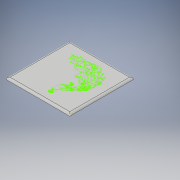
# Autodesk Inventor part: Card_1
Saved by Autodesk Inventor 2019.4 (Build 234330000, 330)
## iProperties
Created: 2020-03-24
Part Number: Card_1
Material: Generic
Document SubType Name: Modeling
Designer: Jorian Brusind
Density: 1 g/cm^3
Appearance: Default
Author: Jorian Brusind
Autodesk Inventor part; units mm, degrees
(part 1 of 2)
ref_plane "YZ Plane" through (0, 0, 0) normal (1, 0, 0) x (0, 1, 0)
ref_plane "XZ Plane" through (0, 0, 0) normal (0, 1, 0) x (-1, 0, 0)
ref_plane "XY Plane" through (0, 0, 0) normal (0, 0, 1) x (1, 0, 0)
sketch "Sketch1" plane through (0, 0, 0) normal (0, 1, 0) x (-1, 0, 0)
  line L0 (0, 0) -> (80, 0)
  line L1 (80, 0) -> (80, -80)
  line L2 (80, -80) -> (0, -80)
  line L3 (0, -80) -> (0, 0)
  line L4 (70, -70) -> (70, -10)
  line L5 (70, -10) -> (10, -10)
  line L6 (10, -10) -> (10, -70)
  line L7 (10, -70) -> (70, -70)
  dimension "d0" = 80
  dimension "d1" = 80
  dimension "d2" = 10
  constraints: 16 end point, 4 parallel, 2 perpendicular, 1 horizontal, 3 other
  measures "d0" distance of L1.end L2.end
  measures "d1" distance of L0.end L1.end
  measures "d2" distance between parallel lines of L1 L4
extrude "Extrusion1" add sketch "Sketch1" along normal blind 2.5
fillet "Fillet1" radius 2.5 4 edges at (-40, 2.5, 0) (0, 2.5, -40) (-40, 2.5, -80) (-80, 2.5, -40)
sketch "Sketch2" plane through (0, 2.5, 0) normal (0, 1, 0) x (1, 0, 0)
  line L0 (-70, 70) -> (-70, 10) projected
  line L1 (-70, 10) -> (-10, 10) projected
  line L2 (-70, 70) -> (-10, 70)
  line L3 (-10, 70) -> (-10, 10)
  line L4 (-10, 10) -> (-70, 10)
  line L5 (-70, 10) -> (-70, 70)
  point P0 (0, 0)
  constraints: 8 end point, 2 parallel, 1 horizontal, 1 perpendicular
extrude "Extrusion2" add sketch "Sketch2" against normal blind 1
sketch "Sketch3" plane through (0, 1.5, 0) normal (0, -1, 0) x (1, 0, 0)
  line L0 (-63.3517, -10.3054) -> (-12.5932, -10.3054) construction
  line L1 (-12.5932, -10.3054) -> (-12.5932, -69.5003) construction
  line L2 (-12.5932, -69.5003) -> (-63.3517, -69.5003) construction
  line L3 (-63.3517, -69.5003) -> (-63.3517, -10.3054) construction
  circle A0 centre (-36.5711, -14.8755) radius 0.2923
  spline S0 degree 4 poles (-35.324, -13.1457) (-35.5446, -13.3836) (-34.7422, -13.6925) (-35.8936, -14.24) (-35.5511, -14.8191) (-35.9597, -15.77) (-36.825, -15.6199) (-37.3254, -15.6398) knots 0 0 0 0 0 0.31317 0.445072 0.586813 1 1 1 1 1
  spline S1 degree 4 poles (-37.3254, -15.6398) (-37.2583, -15.4035) (-36.9842, -15.1648) (-37.3716, -13.9172) (-35.5713, -13.5514) (-35.7305, -13.4977) (-36.1286, -13.2161) knots 0 0 0 0 0 0.420009 0.598576 1 1 1 1 1
  spline S2 degree 4 poles (-36.1286, -13.2161) (-36.1977, -13.1672) (-36.3236, -13.3314) (-37.1252, -12.6262) (-37.6158, -14.3916) (-38.3336, -14.3814) (-38.1098, -15.4286) knots 0 0 0 0 0 0.20425 0.384643 1 1 1 1 1
  spline S3 degree 3 poles (-38.9144, -17.1685) (-39.2781, -16.9978) (-37.8451, -15.6043) (-38.1098, -15.4286) knots 0 0 0 0 1 1 1 1
  spline S4 degree 4 poles (-38.9144, -17.1685) (-38.8152, -17.5134) (-37.7404, -15.2772) (-37.1183, -18.5822) (-34.1569, -13.527) (-35.4039, -17.8434) (-35.7063, -17.3998) knots 0 0 0 0 0 0.380958 0.551634 1 1 1 1 1
  spline S5 degree 4 poles (-35.324, -13.1457) (-35.5269, -12.7152) (-30.8309, -14.436) (-33.9129, -18.4293) (-33.8615, -18.3326) knots 0 0 0 0 0 1 1 1 1 1
  spline S6 degree 4 poles (-33.8615, -18.3326) (-35.1288, -18.3656) (-31.8331, -20.408) (-33.8396, -20.6327) (-27.0068, -23.04) (-26.7008, -23.4984) (-25.4635, -25.0323) (-25.2341, -25.4897) knots 0 0 0 0 0 0.314732 0.481412 0.642299 1 1 1 1 1
  spline S7 degree 4 poles (-25.2341, -25.4897) (-25.4023, -25.6156) (-25.7938, -24.9389) (-27.0573, -23.6199) (-30.4827, -22.3618) (-31.9985, -23.0805) (-32.4743, -21.943) (-37.6197, -21.044) (-37.7605, -24.854) (-36.5634, -26.7006) (-35.7063, -26.8823) knots 0 0 0 0 0 0.17093 0.27416 0.381186 0.49379 0.600301 0.71651 1 1 1 1 1
  spline S8 degree 4 poles (-35.7063, -26.8823) (-35.4306, -26.8662) (-35.7103, -27.6356) (-37.8889, -26.2872) (-36.9937, -25.7229) (-38.9297, -25.107) (-37.7887, -22.8322) (-39.896, -21.88) (-38.051, -17.7127) (-36.0866, -18.5751) (-35.7063, -17.3998) knots 0 0 0 0 0 0.15712 0.241782 0.341646 0.440215 0.558312 0.68699 1 1 1 1 1
  spline S9 degree 5 poles (-33.3611, -22.4991) (-33.2761, -22.525) (-33.1323, -22.7463) (-33.0805, -23.4713) (-31.2722, -23.0711) (-30.0002, -22.6532) (-27.8482, -26.1645) (-29.0106, -24.5854) (-29.6261, -24.0335) (-30.7533, -23.6216) (-31.6668, -24.1266) (-33.7566, -23.2068) (-33.5906, -22.5757) (-33.4394, -22.4753) (-33.3611, -22.4991) knots 0 0 0 0 0 0 0.106127 0.195486 0.298213 0.408816 0.518685 0.625012 0.727572 0.824846 0.902338 1 1 1 1 1 1
  spline S10 degree 4 poles (-34.5544, -27.0158) (-34.756, -26.8509) (-32.4655, -27.7887) (-33.815, -25.1287) (-31.1635, -27.2727) (-31.4203, -24.5805) (-29.3028, -26.5518) (-30.6351, -24.5794) (-28.6311, -25.5338) knots 0 0 0 0 0 0.293192 0.431361 0.562283 0.684411 1 1 1 1 1
  spline S11 degree 4 poles (-28.6311, -25.5338) (-28.4787, -25.3926) (-28.0839, -26.0174) (-29.7828, -25.7606) (-29.7026, -26.1515) (-30.1461, -26.5172) (-30.7038, -26.0429) (-30.8578, -26.9801) (-31.5435, -26.9955) (-31.992, -27.4243) (-32.6157, -26.6422) (-32.7974, -28.0141) (-33.9737, -27.5055) (-34.4403, -27.4572) (-34.5544, -27.0158) knots 0 0 0 0 0 0.143761 0.210775 0.282047 0.347044 0.419443 0.494672 0.570855 0.64562 0.720443 0.799389 1 1 1 1 1
  spline S12 degree 3 poles (-32.3859, -20.0818) (-31.8556, -19.6395) (-27.7329, -20.2333) (-26.6799, -22.7987) knots 0 0 0 0 1 1 1 1
  spline S13 degree 4 poles (-32.3859, -20.0818) (-32.544, -20.1533) (-29.582, -22.2131) (-29.798, -20.0561) (-26.6184, -23.2562) (-26.6799, -22.7987) knots 0 0 0 0 0 0.510331 1 1 1 1 1
  spline S14 degree 4 poles (-35.9258, -27.4345) (-35.5506, -27.1339) (-35.543, -28.1757) (-33.3169, -27.6119) (-32.9054, -28.5495) (-32.099, -29.7207) (-30.6072, -30.9729) (-29.9615, -30.1066) (-29.5156, -30.5716) knots 0 0 0 0 0 0.273602 0.406043 0.548907 0.683354 1 1 1 1 1
  spline S15 degree 4 poles (-29.5156, -30.5716) (-29.2202, -30.6478) (-30.1433, -31.6427) (-30.3254, -30.3824) (-31.1214, -31.3006) (-30.8679, -31.6024) (-30.842, -32.4055) (-30.1008, -32.916) (-30.8967, -33.4395) (-30.1082, -33.9699) (-29.7346, -34.3371) knots 0 0 0 0 0 0.231424 0.328427 0.428678 0.530661 0.628034 0.725923 1 1 1 1 1
  spline S16 degree 4 poles (-29.7346, -34.3371) (-29.3878, -34.6781) (-30.3659, -34.1189) (-30.4227, -34.2157) (-31.503, -34.2428) (-31.5893, -34.4521) (-33.027, -35.5237) (-32.9708, -34.6703) (-31.8667, -34.1719) (-32.5619, -34.097) (-32.7749, -34.3573) (-33.9131, -34.6609) (-33.5335, -33.9376) (-33.0108, -34.1956) (-32.4249, -33.8451) (-32.9337, -33.674) (-33.706, -33.5322) (-32.7473, -33.2202) (-32.3814, -33.4344) (-31.5548, -33.5668) (-31.3728, -33.9075) (-31.1352, -33.3806) knots 0 0 0 0 0 0.102598 0.152726 0.207977 0.263777 0.320477 0.373024 0.41872 0.467777 0.51215 0.561575 0.609015 0.651576 0.696303 0.740357 0.785856 0.834092 0.882144 1 1 1 1 1
  spline S17 degree 4 poles (-31.1352, -33.3806) (-31.1314, -33.1006) (-31.0926, -32.3796) (-31.5407, -32.0448) (-31.6958, -30.9795) knots 0 0 0 0 0 1 1 1 1 1
  spline S18 degree 4 poles (-31.6958, -30.9795) (-31.666, -30.9185) (-32.9258, -29.9607) (-33.0237, -28.6807) (-34.4784, -28.818) (-36.393, -27.4471) (-35.9258, -27.4345) knots 0 0 0 0 0 0.400646 0.601925 1 1 1 1 1
  spline S19 degree 4 poles (-32.5781, -28.1533) (-32.0733, -28.1334) (-32.5286, -29.7003) (-28.3942, -29.6937) (-27.0116, -29.0351) (-27.4794, -30.2319) knots 0 0 0 0 0 0.455262 1 1 1 1 1
  spline S20 degree 4 poles (-32.5781, -28.1533) (-32.752, -28.8754) (-30.7966, -29.9892) (-29.2732, -30.7108) (-27.4794, -30.2319) knots 0 0 0 0 0 1 1 1 1 1
  spline S21 degree 3 poles (-31.9981, -27.8266) (-31.3048, -28.2374) (-30.1278, -28.9395) (-28.02, -28.4008) knots 0 0 0 0 1 1 1 1
  spline S22 degree 3 poles (-31.9981, -27.8266) (-32.159, -28.3516) (-29.309, -29.8112) (-26.2551, -28.9797) knots 0 0 0 0 1 1 1 1
  spline S23 degree 3 poles (-28.02, -28.4008) (-27.4223, -28.5754) (-26.0857, -27.8191) (-26.2551, -28.9797) knots 0 0 0 0 1 1 1 1
  spline S24 degree 5 poles (-30.8304, -27.4166) (-30.8198, -27.3784) (-30.735, -27.3314) (-30.4283, -27.377) (-30.3728, -27.806) (-29.4819, -27.5359) (-28.6522, -28.0829) (-26.9449, -27.1371) (-26.9592, -28.3103) (-27.5005, -27.9622) (-28.3391, -28.2269) (-29.6001, -27.9856) (-29.9402, -28.0264) (-30.7153, -27.6691) (-30.8488, -27.4824) (-30.8304, -27.4166) knots 0 0 0 0 0 0 0.06847 0.134935 0.226492 0.320983 0.41447 0.511985 0.607211 0.700225 0.797172 0.882041 1 1 1 1 1 1
  spline S25 degree 5 poles (-29.6277, -27.2599) (-29.6131, -27.1962) (-29.3962, -27.1169) (-28.6593, -27.1471) (-28.6951, -27.3926) (-26.953, -26.1162) (-27.3022, -26.7784) (-25.8648, -27.2556) (-26.7786, -27.9342) (-26.8765, -27.0905) (-27.6032, -27.0829) (-28.3562, -27.7093) (-29.4112, -27.4986) (-29.6452, -27.3368) (-29.6277, -27.2599) knots 0 0 0 0 0 0 0.117746 0.200054 0.303318 0.403009 0.497632 0.581512 0.677264 0.774 0.857863 1 1 1 1 1 1
  spline S26 degree 5 poles (-28.9567, -26.8367) (-28.8039, -26.8311) (-28.3186, -26.542) (-27.1771, -25.5262) (-25.4527, -27.3948) (-24.9989, -26.5696) (-26.8849, -25.2773) (-28.7538, -25.9258) (-29.1284, -26.6777) (-29.0748, -26.841) (-28.9567, -26.8367) knots 0 0 0 0 0 0 0.223292 0.365456 0.553127 0.712011 0.827339 1 1 1 1 1 1
  spline S27 degree 5 poles (-25.2341, -24.8772) (-25.2139, -24.9767) (-25.0028, -25.1808) (-24.3449, -25.5142) (-25.0904, -26.3444) (-23.5868, -25.9629) (-22.7451, -26.6919) (-21.7421, -27.7341) (-22.2449, -26.4551) (-23.5022, -25.9794) (-23.9866, -24.5416) (-25.0568, -24.5977) (-25.2586, -24.7561) (-25.2341, -24.8772) knots 0 0 0 0 0 0 0.119065 0.209319 0.316618 0.415827 0.527874 0.652848 0.762595 0.855295 1 1 1 1 1 1
  spline S28 degree 3 poles (-23.9961, -26.7161) (-22.4627, -27.8802) (-20.8684, -31.6059) (-18.6876, -30.7743) knots 0 0 0 0 1 1 1 1
  spline S29 degree 4 poles (-23.9961, -26.7161) (-23.918, -26.6354) (-22.7506, -26.261) (-21.1004, -29.3277) (-20.4862, -29.8276) (-19.4071, -30.9349) (-18.4206, -30.3496) (-18.6876, -30.7743) knots 0 0 0 0 0 0.362224 0.54379 0.715209 1 1 1 1 1
  spline S30 degree 5 poles (-23.9961, -27.4166) (-24.0084, -27.3157) (-23.7565, -27.4117) (-22.6333, -28.3225) (-21.0445, -30.8303) (-20.9846, -30.4847) (-22.2092, -31.6756) (-21.8204, -30.0675) (-22.8853, -29.6975) (-22.7683, -28.9575) (-23.686, -27.943) (-23.9837, -27.5186) (-23.9961, -27.4166) knots 0 0 0 0 0 0 0.168899 0.268082 0.386273 0.508516 0.61038 0.728446 0.829264 1 1 1 1 1 1
  spline S31 degree 3 poles (-24.0993, -28.03) (-23.4446, -28.7383) (-20.4539, -32.1956) (-23.4494, -35.6288) knots 0 0 0 0 1 1 1 1
  spline S32 degree 4 poles (-23.4494, -35.6288) (-24.264, -35.9348) (-24.9335, -34.8994) (-23.1097, -35.9947) (-21.6779, -30.0877) (-24.1929, -28.6957) (-24.0993, -28.03) knots 0 0 0 0 0 0.300614 0.469562 1 1 1 1 1
  spline S33 degree 4 poles (-25.0725, -27.5346) (-24.8746, -27.2275) (-22.7058, -29.9805) (-23.1973, -34.4136) (-26.2584, -32.3924) (-25.4951, -32.4837) (-23.7291, -31.7895) (-24.1652, -30.0658) (-23.9832, -28.6385) (-25.4514, -27.5272) (-25.0725, -27.5346) knots 0 0 0 0 0 0.306197 0.41617 0.507229 0.595458 0.6902 0.801188 1 1 1 1 1
  spline S34 degree 5 poles (-25.9194, -27.3048) (-25.9589, -27.3397) (-25.8277, -27.6124) (-25.1566, -28.4149) (-25.287, -28.3236) (-24.9688, -32.2896) (-27.6153, -30.4366) (-26.2254, -32.3751) (-25.0718, -30.9028) (-24.5869, -30.5734) (-24.0451, -29.0091) (-25.4585, -27.5295) (-25.8674, -27.2588) (-25.9194, -27.3048) knots 0 0 0 0 0 0 0.120573 0.208552 0.309906 0.418809 0.526835 0.630512 0.742533 0.841179 1 1 1 1 1 1
  ellipse E0 centre (-21.017, -31.7834) end of major axis (-21.2816, -31.2172) minor radius 0.4541
  ellipse E1 centre (-18.4895, -33.3373) end of major axis (-18.8637, -32.8075) minor radius 0.4897
  ellipse E2 centre (-21.6934, -42.4408) end of major axis (-21.1885, -41.4828) minor radius 0.8739
  ellipse E3 centre (-15.5478, -42.5952) end of major axis (-15.5478, -41.4335) minor radius 0.8581
  ellipse E4 centre (-19.3699, -49.1886) end of major axis (-18.9081, -47.7943) minor radius 1.306
  ellipse E5 centre (-27.7073, -52.7002) end of major axis (-26.5866, -51.7716) minor radius 1.2181
  ellipse E6 centre (-17.1812, -55.9206) end of major axis (-16.5391, -54.5789) minor radius 0.9936
  ellipse E7 centre (-28.8439, -61.7728) end of major axis (-27.7073, -61.3217) minor radius 0.7832
  ellipse E8 centre (-44.2997, -60.5199) end of major axis (-42.6078, -60.5199) minor radius 1.1489
  spline S35 degree 3 poles (-19.5271, -31.3956) (-19.0196, -31.8926) (-17.7371, -31.8552) (-17.9516, -31.0393) knots 0 0 0 0 1 1 1 1
  spline S36 degree 4 poles (-17.9516, -31.0393) (-17.8718, -30.4122) (-15.8826, -33.3458) (-19.1868, -32.8117) (-19.5271, -31.3956) knots 0 0 0 0 0 1 1 1 1 1
  spline S37 degree 4 poles (-20.8379, -34.6217) (-19.4947, -34.9164) (-21.2318, -32.5629) (-17.6677, -33.2688) (-20.3107, -30.9795) knots 0 0 0 0 0 1 1 1 1 1
  spline S38 degree 4 poles (-20.3107, -30.9795) (-20.6685, -30.6769) (-20.6934, -31.3689) (-19.9364, -31.3263) (-20.195, -32.8112) (-20.9449, -32.9065) (-21.6592, -32.7466) (-21.7848, -31.827) (-21.907, -31.6466) knots 0 0 0 0 0 0.267734 0.396357 0.532031 0.670594 1 1 1 1 1
  spline S39 degree 4 poles (-21.907, -31.6466) (-22.3419, -31.4487) (-20.8709, -33.7898) (-21.5359, -33.7291) (-21.2111, -34.7898) (-20.8379, -34.6217) knots 0 0 0 0 0 0.51757 1 1 1 1 1
  spline S40 degree 4 poles (-20.766, -35.1172) (-19.8876, -34.9373) (-20.1572, -33.9627) (-19.4524, -34.5635) (-19.7247, -36.2501) (-20.5302, -36.787) (-21.0324, -36.7624) (-21.7811, -36.3233) (-21.8838, -35.5783) (-22.1093, -35.1229) (-21.5483, -33.5183) (-21.5122, -35.2087) (-21.2854, -35.0098) (-20.766, -35.1172) knots 0 0 0 0 0 0.182152 0.257602 0.342773 0.433832 0.515997 0.595919 0.678531 0.753704 0.825493 1 1 1 1 1
  spline S41 degree 4 poles (-19.0268, -34.0685) (-18.7409, -34.1417) (-17.1836, -35.7942) (-17.1543, -32.9167) (-17.764, -32.9276) knots 0 0 0 0 0 1 1 1 1 1
  spline S42 degree 4 poles (-17.764, -32.9276) (-17.8387, -32.6933) (-17.3458, -32.89) (-16.8285, -33.1066) (-16.4625, -33.8615) (-16.5379, -34.5141) (-16.7185, -35.0701) (-17.2038, -35.2058) (-17.6314, -35.4748) (-18.4579, -35.193) (-18.9875, -34.8196) (-19.2024, -34.218) (-19.0268, -34.0685) knots 0 0 0 0 0 0.171381 0.262578 0.355555 0.445026 0.530668 0.614709 0.701973 0.792644 1 1 1 1 1
  spline S43 degree 5 poles (-19.4194, -35.9625) (-19.295, -36.0313) (-18.9705, -36.0406) (-18.3013, -35.7473) (-19.0957, -35.6603) (-18.9284, -34.9173) (-19.3485, -34.7866) (-19.4737, -33.2171) (-19.6394, -35.2858) (-19.2948, -35.023) (-19.6406, -35.6443) (-19.5523, -35.8889) (-19.4194, -35.9625) knots 0 0 0 0 0 0 0.143801 0.239764 0.360191 0.482966 0.611681 0.742234 0.846271 1 1 1 1 1 1
  spline S44 degree 5 poles (-14.3221, -37.2251) (-14.273, -37.225) (-14.2224, -37.0537) (-14.2438, -36.3783) (-14.2395, -36.1076) (-14.5116, -35.2835) (-14.6889, -34.9296) (-15.1743, -34.5084) (-15.5757, -34.3933) (-16.2251, -34.3778) (-16.6103, -34.6493) (-15.7195, -35.1067) (-15.4355, -35.1895) (-14.7936, -36.0142) (-14.7853, -36.1341) (-14.5112, -37.0079) (-14.3779, -37.2252) (-14.3221, -37.2251) knots 0 0 0 0 0 0 0.092663 0.155941 0.233987 0.313281 0.389538 0.457583 0.525214 0.594431 0.66685 0.742099 0.825589 0.894681 1 1 1 1 1 1
  spline S45 degree 5 poles (-16.4214, -35.3061) (-16.4018, -35.2543) (-16.2185, -35.2898) (-15.5483, -35.7263) (-15.4414, -36.4002) (-14.5668, -37.0976) (-13.8258, -38.4064) (-14.0517, -39.8851) (-13.261, -40.9923) (-14.3695, -42.258) (-12.1945, -43.4637) (-13.432, -43.6748) (-13.7621, -42.6858) (-14.2319, -42.0616) (-14.6289, -41.0906) (-15.0867, -39.8382) (-14.7116, -38.763) (-15.4988, -37.4661) (-15.0187, -36.9438) (-16.2114, -35.7589) (-16.45, -35.3819) (-16.4214, -35.3061) knots 0 0 0 0 0 0 0.053732 0.097834 0.156445 0.222119 0.289791 0.356859 0.415576 0.469792 0.521624 0.571562 0.623429 0.682083 0.742885 0.805694 0.870231 0.921522 1 1 1 1 1 1
  spline S46 degree 5 poles (-15.9677, -40.9926) (-15.8484, -41.0734) (-15.4979, -41.1314) (-14.658, -40.9692) (-15.504, -40.7181) (-15.1203, -39.5113) (-15.3578, -39.0368) (-15.735, -37.7705) (-15.5769, -38.0538) (-16.6952, -35.2921) (-16.4608, -36.6677) (-16.3319, -36.6643) (-16.0555, -37.7254) (-16.253, -38.0379) (-15.8485, -38.8772) (-16.2821, -39.9553) (-15.7901, -40.2184) (-16.1432, -40.7024) (-16.0829, -40.9145) (-15.9677, -40.9926) knots 0 0 0 0 0 0 0.07587 0.12937 0.197561 0.265254 0.343498 0.415321 0.482169 0.547672 0.611 0.670605 0.737417 0.806106 0.872412 0.926727 1 1 1 1 1 1
  spline S47 degree 5 poles (-17.6207, -41.3723) (-17.526, -41.4325) (-17.2108, -41.1854) (-16.3758, -39.8158) (-16.2257, -40.0312) (-16.9062, -34.882) (-17.3821, -36.4562) (-16.7825, -37.4206) (-17.3208, -38.3171) (-17.1453, -39.4507) (-17.3233, -39.9427) (-17.5615, -40.3444) (-17.719, -41.0919) (-17.6859, -41.3309) (-17.6207, -41.3723) knots 0 0 0 0 0 0 0.141772 0.233793 0.345818 0.460441 0.567888 0.654576 0.746613 0.834588 0.902411 1 1 1 1 1 1
  spline S48 degree 5 poles (-18.9081, -36.4109) (-18.8365, -36.4058) (-18.7132, -36.2971) (-18.505, -35.8809) (-18.0681, -37.0072) (-18.3049, -37.1322) (-18.62, -37.8454) (-19.0368, -37.7127) (-19.4634, -37.4155) (-19.5131, -36.9259) (-19.5161, -36.4286) (-19.2378, -36.0701) (-19.069, -36.3536) (-18.9668, -36.4151) (-18.9081, -36.4109) knots 0 0 0 0 0 0 0.122221 0.208647 0.312805 0.419979 0.526064 0.631352 0.728714 0.824557 0.89992 1 1 1 1 1 1
  spline S49 degree 5 poles (-19.868, -37.2702) (-19.7939, -37.2817) (-19.7018, -37.5036) (-19.6382, -38.2929) (-18.9612, -38.4002) (-18.6891, -38.4019) (-17.5038, -37.8134) (-18.2743, -37.0477) (-17.5089, -36.693) (-17.6449, -37.7812) (-17.2851, -37.9782) (-17.5203, -39.0215) (-18.0572, -39.4942) (-18.7508, -39.8247) (-19.5524, -39.6958) (-20.0798, -38.9816) (-20.5418, -38.6362) (-20.1437, -37.5098) (-19.9557, -37.2566) (-19.868, -37.2702) knots 0 0 0 0 0 0 0.079097 0.133351 0.199973 0.259999 0.31817 0.376815 0.434654 0.494724 0.561731 0.630756 0.701479 0.773466 0.846774 0.906384 1 1 1 1 1 1
  spline S50 degree 5 poles (-20.6923, -37.0413) (-20.7937, -37.0047) (-21.0413, -36.9685) (-21.5325, -37.0126) (-20.8933, -38.8414) (-21.5679, -38.581) (-23.2741, -41.9479) (-21.3958, -39.6024) (-21.2051, -41.2401) (-19.7575, -40.5302) (-20.431, -38.9723) (-20.3653, -38.4828) (-20.4975, -37.3272) (-20.4955, -37.1504) (-20.6075, -37.0719) (-20.6923, -37.0413) knots 0 0 0 0 0 0 0.097411 0.176594 0.273172 0.374402 0.47305 0.572074 0.667248 0.76187 0.848421 0.918566 1 1 1 1 1 1
  spline S51 degree 5 poles (-22.7021, -36.6766) (-22.6255, -36.6777) (-22.6974, -37.1269) (-23.3882, -38.9246) (-23.5146, -38.9014) (-25.1864, -40.3908) (-26.3321, -39.047) (-25.6333, -37.8786) (-25.2484, -39.3618) (-23.512, -38.3052) (-23.7144, -38.3107) (-23.0402, -37.0298) (-22.771, -36.6757) (-22.7021, -36.6766) knots 0 0 0 0 0 0 0.15502 0.255703 0.369442 0.475363 0.577682 0.674868 0.774185 0.860446 1 1 1 1 1 1
  spline S52 degree 5 poles (-25.9194, -39.9564) (-25.8568, -39.8675) (-25.6947, -39.7741) (-25.3735, -39.8915) (-25.178, -40.5024) (-24.1491, -40.6864) (-23.3894, -38.3827) (-23.1178, -39.7388) (-23.788, -40.0679) (-24.3296, -41.0394) (-25.1127, -41.0528) (-25.8923, -40.9387) (-26.0618, -40.3521) (-25.9966, -40.0659) (-25.9194, -39.9564) knots 0 0 0 0 0 0 0.097167 0.178472 0.272394 0.374095 0.481458 0.588908 0.688995 0.795073 0.880225 1 1 1 1 1 1
  spline S53 degree 5 poles (-23.6773, -40.4903) (-23.7403, -40.4915) (-24.0697, -40.8192) (-24.9394, -42.0181) (-25.2947, -41.9445) (-28.8609, -41.9407) (-26.1114, -38.825) (-26.8434, -38.3736) (-28.4707, -39.4153) (-29.0191, -40.5968) (-29.1007, -42.1233) (-28.5038, -43.7786) (-25.2936, -43.2241) (-23.8074, -41.0011) (-23.595, -40.4888) (-23.6773, -40.4903) knots 0 0 0 0 0 0 0.100514 0.176245 0.26015 0.345845 0.430864 0.512875 0.589614 0.68684 0.786528 0.868762 1 1 1 1 1 1
  spline S54 degree 5 poles (-24.6908, -42.4408) (-24.6752, -42.393) (-25.0601, -42.737) (-26.8708, -44.1831) (-31.9957, -42.5107) (-28.2661, -40.9249) (-31.6416, -41.4215) (-30.0509, -43.6668) (-29.5125, -45.0219) (-27.3191, -43.7658) (-26.0983, -44.2645) (-25.0405, -42.8697) (-24.7038, -42.4807) (-24.6908, -42.4408) knots 0 0 0 0 0 0 0.158055 0.24384 0.351874 0.456147 0.552268 0.661577 0.775793 0.867758 1 1 1 1 1 1
  spline S55 degree 5 poles (-25.2341, -43.4317) (-25.1924, -43.4992) (-25.5014, -43.9313) (-26.8993, -45.2825) (-26.7325, -44.4638) (-30.1181, -47.5213) (-32.5025, -44.406) (-32.3496, -45.0895) (-31.9495, -42.1318) (-31.5883, -45.7921) (-29.934, -44.6823) (-28.3721, -44.9415) (-27.5605, -44.8505) (-25.7665, -43.5789) (-25.2789, -43.3592) (-25.2341, -43.4317) knots 0 0 0 0 0 0 0.110426 0.194056 0.289831 0.381901 0.471538 0.551049 0.627069 0.712229 0.804571 0.88137 1 1 1 1 1 1
  spline S56 degree 4 poles (-16.7028, -41.7671) (-16.7718, -42.0891) (-17.666, -43.0083) (-16.1263, -45.859) (-13.3331, -43.0811) (-14.7803, -41.8234) (-14.3414, -41.8665) knots 0 0 0 0 0 0.426284 0.626921 1 1 1 1 1
  spline S57 degree 4 poles (-16.7028, -41.7671) (-16.6641, -41.5106) (-17.9576, -41.6654) (-18.6674, -44.605) (-16.0179, -46.1328) (-14.9085, -45.9068) (-13.8194, -45.0981) (-13.2798, -43.4716) (-14.0576, -42.9903) (-14.1007, -41.8543) (-14.3414, -41.8665) knots 0 0 0 0 0 0.222739 0.348409 0.478006 0.595308 0.697659 0.798062 1 1 1 1 1
  spline S58 degree 5 poles (-21.9665, -45.663) (-21.655, -45.6435) (-21.192, -45.5086) (-20.6379, -45.2176) (-19.0128, -44.1353) (-20.1961, -40.7197) (-20.3046, -42.6102) (-20.3673, -43.3526) (-21.5157, -44.0797) (-21.8325, -44.1136) (-22.8924, -43.8727) (-22.7508, -43.2466) (-23.2761, -42.3972) (-22.3449, -41.9248) (-23.0675, -41.3778) (-23.2882, -42.915) (-23.8087, -42.7872) (-23.6321, -45.1617) (-22.8076, -45.6142) (-22.2748, -45.6823) (-21.9665, -45.663) knots 0 0 0 0 0 0 0.096451 0.156987 0.230609 0.303506 0.366259 0.423266 0.480107 0.535632 0.587827 0.635381 0.682364 0.730983 0.786628 0.848109 0.904537 1 1 1 1 1 1
  spline S59 degree 4 poles (-22.2381, -36.4531) (-22.8148, -37.4509) (-22.4915, -41.0288) (-26.7342, -46.1859) (-31.2126, -50.8947) (-39.0632, -48.6536) (-37.1125, -44.3644) (-36.2885, -43.7981) (-34.6877, -43.6821) (-34.1216, -44.7104) (-34.7241, -45.668) (-35.7723, -45.5331) (-36.0279, -44.7718) (-36.2295, -44.7971) knots 0 0 0 0 0 0.254923 0.381002 0.50238 0.603921 0.687075 0.750992 0.803574 0.853542 0.90037 1 1 1 1 1
  spline S60 degree 4 poles (-36.2295, -44.7971) (-36.3319, -44.4655) (-38.4253, -46.8518) (-33.2322, -47.508) (-33.0156, -44.8927) (-34.3601, -43.0701) (-36.7113, -42.9821) (-38.2662, -44.3442) (-39.4356, -45.6692) (-38.513, -48.5141) (-37.239, -49.9573) (-35.6171, -51.1801) (-32.3398, -50.9628) (-29.0415, -49.8873) (-25.2886, -46.4884) (-23.7716, -43.6888) (-22.1989, -39.2047) (-22.0879, -36.7399) (-22.2381, -36.4531) knots 0 0 0 0 0 0.099125 0.150623 0.204522 0.255952 0.307635 0.361124 0.414483 0.467234 0.523479 0.583259 0.650298 0.721512 0.796232 0.86839 1 1 1 1 1
  spline S61 degree 5 poles (-18.9081, -40.2818) (-18.9562, -40.2762) (-18.9414, -40.7194) (-18.6683, -42.4586) (-19.2107, -43.0885) (-18.3331, -44.915) (-20.2426, -47.7474) (-18.9914, -47.094) (-17.9933, -47.8826) (-18.5344, -45.8552) (-17.992, -44.3262) (-18.4671, -44.1209) (-18.1572, -42.7039) (-18.6723, -40.774) (-18.8574, -40.2877) (-18.9081, -40.2818) knots 0 0 0 0 0 0 0.115426 0.198588 0.293846 0.385315 0.4713 0.552712 0.625691 0.708342 0.801754 0.878266 1 1 1 1 1 1
  spline S62 degree 5 poles (-22.0581, -46.5929) (-22.1637, -46.5881) (-22.4574, -47.1397) (-23.0877, -49.3043) (-23.1947, -49.3009) (-27.5999, -53.7516) (-24.1126, -52.5565) (-23.0947, -50.468) (-22.2082, -49.4152) (-21.8976, -47.1486) (-21.9538, -46.5976) (-22.0581, -46.5929) knots 0 0 0 0 0 0 0.169901 0.281259 0.42469 0.578913 0.723423 0.832185 1 1 1 1 1 1
  spline S63 degree 5 poles (-27.3781, -49.9393) (-27.359, -50.0363) (-26.953, -49.9522) (-25.4766, -49.2349) (-25.1581, -49.0955) (-22.8644, -45.2547) (-23.9099, -45.0525) (-24.0848, -46.7652) (-25.4888, -47.9794) (-25.592, -48.2765) (-27.0332, -49.4252) (-27.3976, -49.8405) (-27.3781, -49.9393) knots 0 0 0 0 0 0 0.15885 0.255617 0.374566 0.502928 0.624081 0.734989 0.838222 1 1 1 1 1 1
  spline S64 degree 5 poles (-17.5715, -49.4488) (-17.6032, -49.4516) (-17.7155, -49.7476) (-18.0546, -50.931) (-18.4571, -51.5975) (-20.4227, -52.0569) (-20.7558, -51.3423) (-22.2558, -50.4765) (-20.2246, -47.9846) (-21.541, -47.9258) (-22.3213, -49.6742) (-22.7302, -50.2884) (-23.4533, -53.4946) (-20.739, -54.0701) (-19.3458, -53.6782) (-17.623, -51.9062) (-17.6917, -50.9703) (-17.5439, -49.7218) (-17.5415, -49.4462) (-17.5715, -49.4488) knots 0 0 0 0 0 0 0.071858 0.121262 0.184103 0.2529 0.313296 0.372498 0.433983 0.499749 0.566342 0.642968 0.72336 0.805515 0.876909 0.931897 1 1 1 1 1 1
  spline S65 degree 5 poles (-17.8243, -52.8158) (-17.7281, -52.8482) (-17.3446, -52.6758) (-16.304, -51.8465) (-15.9294, -51.8749) (-15.5762, -48.1065) (-15.1115, -47.3367) (-15.1519, -45.8197) (-16.0099, -47.8116) (-16.0467, -48.2537) (-16.1963, -50.0069) (-16.8127, -51.2413) (-17.5749, -52.0482) (-17.9037, -52.6381) (-17.8894, -52.7938) (-17.8243, -52.8158) knots 0 0 0 0 0 0 0.120486 0.208383 0.303313 0.396902 0.48845 0.569784 0.656452 0.754977 0.846156 0.918393 1 1 1 1 1 1
  spline S66 degree 5 poles (-13.1277, -50.2078) (-13.0759, -50.1678) (-13.0525, -49.9379) (-13.2236, -49.1777) (-13.1831, -48.5751) (-13.0255, -47.994) (-13.8098, -44.1369) (-14.013, -46.2614) (-14.4823, -47.4751) (-14.1441, -48.7508) (-13.7794, -49.6012) (-13.3393, -50.171) (-13.178, -50.2467) (-13.1277, -50.2078) knots 0 0 0 0 0 0 0.110172 0.203227 0.312459 0.435631 0.564354 0.695229 0.802174 0.892943 1 1 1 1 1 1
  spline S67 degree 5 poles (-14.7024, -46.8903) (-14.6608, -46.875) (-14.5829, -47.1426) (-14.4797, -48.2905) (-14.3436, -48.685) (-14.0959, -50.8511) (-12.6281, -50.4075) (-12.4652, -51.5113) (-13.3686, -51.9722) (-14.0607, -51.8442) (-14.3719, -50.7801) (-14.78, -50.0554) (-14.5938, -48.9372) (-14.8588, -48.5037) (-14.8106, -47.2404) (-14.7456, -46.9062) (-14.7024, -46.8903) knots 0 0 0 0 0 0 0.102025 0.175223 0.261179 0.34961 0.429431 0.503031 0.576916 0.654641 0.737182 0.82359 0.893795 1 1 1 1 1 1
  spline S68 degree 5 poles (-15.1301, -49.5893) (-15.2022, -49.5308) (-15.2708, -49.9937) (-15.1428, -52.223) (-15.2082, -51.5979) (-15.3695, -55.0901) (-13.255, -54.4102) (-12.867, -51.9396) (-13.8421, -52.6557) (-14.1052, -53.1854) (-15.015, -51.7514) (-14.6738, -51.8598) (-14.9151, -50.1804) (-15.0627, -49.644) (-15.1301, -49.5893) knots 0 0 0 0 0 0 0.138812 0.234837 0.349484 0.455656 0.550192 0.634869 0.712802 0.798155 0.870273 1 1 1 1 1 1
  spline S69 degree 5 poles (-16.4214, -60.807) (-16.507, -60.7917) (-16.7138, -60.8741) (-17.1119, -61.2429) (-17.559, -60.156) (-16.8723, -59.7574) (-15.6493, -58.7254) (-13.9907, -56.5187) (-14.9412, -56.0652) (-15.29, -53.4421) (-15.7741, -54.0854) (-15.219, -50.2913) (-16.3397, -53.409) (-15.94, -54.1818) (-15.4555, -55.3065) (-15.2933, -57.1535) (-16.177, -57.7501) (-17.2727, -59.1159) (-18.3275, -59.4148) (-19.0548, -61.7774) (-16.466, -62.1641) (-16.1918, -61.0566) (-16.307, -60.8276) (-16.4214, -60.807) knots 0 0 0 0 0 0 0.040705 0.074279 0.123063 0.176595 0.235523 0.294986 0.353234 0.405946 0.459071 0.511076 0.566198 0.620286 0.676422 0.732621 0.790623 0.849095 0.903186 0.945553 1 1 1 1 1 1
  spline S70 degree 5 poles (-16.7028, -57.4388) (-16.6468, -57.5035) (-16.8035, -57.8135) (-17.758, -58.8179) (-18.1386, -58.7081) (-19.9023, -58.9013) (-20.5634, -57.8237) (-21.0699, -56.27) (-18.9089, -53.6391) (-16.9047, -54.903) (-19.0155, -54.4617) (-19.2622, -55.9209) (-19.5336, -56.6691) (-19.1671, -57.5038) (-18.3756, -57.893) (-17.9014, -57.9225) (-17.0324, -57.4424) (-16.7529, -57.3809) (-16.7028, -57.4388) knots 0 0 0 0 0 0 0.085763 0.144817 0.223528 0.311824 0.392479 0.469601 0.547007 0.618217 0.678593 0.743324 0.809692 0.873231 0.923311 1 1 1 1 1 1
  spline S71 degree 5 poles (-22.5249, -53.9679) (-22.3913, -53.9936) (-22.4915, -54.5193) (-23.5796, -56.6468) (-23.9037, -58.3303) (-30.7578, -58.919) (-27.145, -58.1965) (-26.8462, -57.6762) (-24.403, -55.9767) (-24.2615, -55.6005) (-23.0864, -54.2818) (-22.6415, -53.9456) (-22.5249, -53.9679) knots 0 0 0 0 0 0 0.159642 0.264441 0.392071 0.529169 0.65311 0.765527 0.860729 1 1 1 1 1 1
  spline S72 degree 5 poles (-27.6912, -56.6247) (-27.722, -56.5194) (-27.1926, -56.1639) (-25.0215, -55.3208) (-26.3914, -56.0485) (-21.4525, -51.5939) (-23.9061, -54.2919) (-23.3004, -54.3027) (-25.3518, -55.9954) (-25.0465, -56.2426) (-27.0963, -56.7247) (-27.6618, -56.725) (-27.6912, -56.6247) knots 0 0 0 0 0 0 0.16177 0.266446 0.390354 0.513343 0.636105 0.75044 0.845764 1 1 1 1 1 1
  spline S73 degree 5 poles (-23.2024, -57.6701) (-23.2994, -57.5784) (-23.1029, -57.1404) (-21.9793, -55.8875) (-22.5017, -56.1094) (-18.6672, -54.1999) (-20.7441, -55.2149) (-20.6854, -56.3751) (-20.9782, -56.6454) (-22.5923, -57.6215) (-23.1038, -57.7634) (-23.2024, -57.6701) knots 0 0 0 0 0 0 0.180126 0.293573 0.432247 0.569126 0.710421 0.816875 1 1 1 1 1 1
  spline S74 degree 5 poles (-26.4343, -53.7933) (-26.5028, -53.7505) (-26.8633, -53.9417) (-27.9992, -54.8939) (-28.8713, -54.6535) (-30.8273, -52.98) (-28.0187, -51.6139) (-28.4027, -50.7404) (-30.2079, -51.8352) (-31.3226, -52.5153) (-31.4815, -54.626) (-30.538, -55.3528) (-29.1744, -55.9746) (-27.7524, -55.5881) (-27.0416, -54.9964) (-26.451, -54.086) (-26.3762, -53.8296) (-26.4343, -53.7933) knots 0 0 0 0 0 0 0.093657 0.161628 0.236101 0.312154 0.388674 0.465048 0.537589 0.620007 0.703667 0.786432 0.861128 0.920616 1 1 1 1 1 1
  spline S75 degree 5 poles (-21.2337, -58.0185) (-21.1413, -58.007) (-21.4532, -58.2528) (-23.1277, -59.2926) (-22.9108, -59.7972) (-24.3608, -61.0863) (-24.3802, -61.8319) (-25.8889, -66.109) (-26.5156, -64.4721) (-24.8775, -63.394) (-26.0108, -61.7004) (-24.3846, -60.6502) (-25.5594, -60.2193) (-22.3064, -58.4846) (-21.3559, -58.0337) (-21.2337, -58.0185) knots 0 0 0 0 0 0 0.100521 0.173126 0.269373 0.358925 0.447092 0.53718 0.620389 0.694446 0.789606 0.867022 1 1 1 1 1 1
  spline S76 degree 5 poles (-22.8953, -64.5283) (-22.8406, -64.557) (-22.6086, -64.3403) (-21.9009, -63.2421) (-21.4289, -63.3251) (-20.9278, -61.1571) (-20.8422, -60.9001) (-19.0045, -58.3235) (-20.874, -59.3012) (-21.4098, -60.8975) (-22.1792, -61.3818) (-22.2034, -63.2823) (-22.5872, -63.3425) (-22.9209, -64.2556) (-22.9427, -64.5034) (-22.8953, -64.5283) knots 0 0 0 0 0 0 0.104275 0.180374 0.276069 0.369888 0.466945 0.562463 0.657102 0.749323 0.840858 0.909515 1 1 1 1 1 1
  spline S77 degree 5 poles (-27.7838, -62.6902) (-27.6387, -62.7251) (-27.7106, -63.1996) (-28.8886, -65.2169) (-30.9613, -65.691) (-33.5447, -63.629) (-32.7448, -62.2102) (-31.9426, -60.2587) (-30.1835, -59.6926) (-27.8066, -60.5921) (-29.9793, -60.491) (-30.8828, -61.0764) (-31.4949, -62.1182) (-31.1136, -63.1411) (-29.8628, -63.4405) (-29.2185, -63.6999) (-28.2863, -62.8731) (-27.8998, -62.6623) (-27.7838, -62.6902) knots 0 0 0 0 0 0 0.098307 0.166497 0.251716 0.342537 0.421441 0.492045 0.561328 0.62589 0.68419 0.745438 0.808705 0.871232 0.921452 1 1 1 1 1 1
  spline S78 degree 5 poles (-26.6799, -63.0975) (-26.8056, -63.1021) (-27.051, -63.551) (-27.4151, -65.4152) (-28.0157, -65.9742) (-29.1354, -66.7087) (-31.1163, -70.56) (-29.1833, -68.0937) (-28.7744, -67.3861) (-26.9111, -66.9986) (-26.688, -65.2731) (-26.2877, -64.5712) (-26.4226, -63.3836) (-26.578, -63.0938) (-26.6799, -63.0975) knots 0 0 0 0 0 0 0.126408 0.214713 0.319295 0.424711 0.528403 0.628408 0.726776 0.822194 0.897538 1 1 1 1 1 1
  spline S79 degree 5 poles (-26.124, -44.9068) (-26.0673, -44.9653) (-26.4441, -45.4473) (-28.5388, -47.2592) (-29.6732, -48.0825) (-31.2783, -48.9341) (-34.8826, -49.0595) (-35.1857, -47.2535) (-32.9666, -45.8904) (-32.9654, -47.6432) (-30.599, -46.7943) (-29.6027, -46.7593) (-27.7821, -46.1271) (-27.3485, -45.5657) (-26.439, -44.9721) (-26.161, -44.8685) (-26.124, -44.9068) knots 0 0 0 0 0 0 0.11821 0.200562 0.297126 0.391341 0.473927 0.552773 0.627933 0.705951 0.785542 0.862498 0.922716 1 1 1 1 1 1
  spline S80 degree 5 poles (-31.1855, -52.0279) (-31.3445, -51.9736) (-31.926, -52.198) (-33.3933, -53.3398) (-34.9658, -51.0852) (-36.5968, -52.6429) (-38.3445, -47.6598) (-38.2869, -52.8398) (-35.9714, -53.2552) (-34.1026, -53.1577) (-31.7045, -53.373) (-31.0414, -52.3501) (-31.0641, -52.0694) (-31.1855, -52.0279) knots 0 0 0 0 0 0 0.135017 0.226539 0.338043 0.455953 0.577488 0.700018 0.808495 0.896992 1 1 1 1 1 1
  spline S81 degree 5 poles (-32.468, -53.8774) (-32.5019, -53.8312) (-32.7767, -53.8616) (-33.7731, -54.2458) (-33.6389, -53.6832) (-35.6781, -54.1135) (-36.1404, -53.36) (-38.7771, -52.8691) (-37.5656, -51.172) (-39.532, -52.4107) (-37.9207, -53.5762) (-37.4189, -54.2872) (-35.7891, -54.9066) (-33.6375, -54.1335) (-33.5479, -54.7744) (-32.5968, -54.1294) (-32.4333, -53.9244) (-32.468, -53.8774) knots 0 0 0 0 0 0 0.078285 0.139807 0.220914 0.299451 0.375836 0.45116 0.52433 0.598906 0.68355 0.771662 0.854885 0.920194 1 1 1 1 1 1
  spline S82 degree 5 poles (-36.2788, -59.6971) (-36.3044, -59.6505) (-35.9955, -59.1657) (-34.5582, -57.2952) (-35.4349, -58.4564) (-29.7912, -54.0122) (-31.6935, -57.0056) (-31.6783, -57.3933) (-33.1565, -58.1631) (-34.977, -58.8753) (-35.3283, -58.8879) (-36.0636, -59.5901) (-36.2617, -59.728) (-36.2788, -59.6971) knots 0 0 0 0 0 0 0.150253 0.251139 0.370905 0.492044 0.614408 0.720857 0.819971 0.900204 1 1 1 1 1 1
  spline S83 degree 5 poles (-33.7839, -55.0647) (-33.8187, -55.002) (-34.461, -55.1737) (-36.8222, -56.1645) (-36.8444, -55.0048) (-42.4902, -54.8791) (-39.8285, -51.7718) (-40.4347, -51.677) (-42.9492, -52.1227) (-43.2201, -52.8336) (-44.0553, -53.6328) (-42.5933, -56.0582) (-41.1368, -55.5266) (-39.2831, -56.686) (-36.7282, -55.8048) (-35.928, -56.404) (-34.1513, -55.4261) (-33.7538, -55.119) (-33.7839, -55.0647) knots 0 0 0 0 0 0 0.097595 0.164169 0.238006 0.313554 0.380948 0.438296 0.496164 0.560935 0.627009 0.699718 0.778514 0.854073 0.915464 1 1 1 1 1 1
  spline S84 degree 5 poles (-35.5982, -56.3935) (-35.6086, -56.296) (-36.3606, -56.3977) (-39.4351, -57.2932) (-40.2202, -57.0034) (-44.9642, -55.8055) (-46.6219, -52.7538) (-42.3616, -51.6147) (-45.4567, -51.6669) (-46.4805, -52.5073) (-47.3733, -53.3033) (-47.5481, -55.7506) (-46.2991, -56.7078) (-44.1509, -57.8502) (-41.8958, -58.1208) (-38.9717, -57.9761) (-38.2444, -57.8) (-36.1147, -56.8167) (-35.5893, -56.4766) (-35.5982, -56.3935) knots 0 0 0 0 0 0 0.091966 0.156155 0.229515 0.30037 0.365122 0.419511 0.472751 0.528675 0.589429 0.653992 0.723149 0.794311 0.865027 0.921643 1 1 1 1 1 1
  spline S85 degree 5 poles (-31.7361, -54.8338) (-31.7561, -54.7996) (-32.3698, -55.0138) (-34.7751, -56.0449) (-35.1452, -56.5542) (-37.9494, -57.7955) (-38.046, -59.4065) (-43.0109, -58.5701) (-41.8576, -59.5823) (-41.8267, -60.0519) (-41.8043, -61.0844) (-39.4135, -59.4859) (-38.1194, -59.3564) (-34.8881, -57.0925) (-34.9179, -56.5609) (-32.3298, -55.2388) (-31.7149, -54.8701) (-31.7361, -54.8338) knots 0 0 0 0 0 0 0.101048 0.173329 0.262138 0.344004 0.414817 0.475042 0.52637 0.580939 0.648797 0.728558 0.816391 0.892782 1 1 1 1 1 1
  spline S86 degree 5 poles (-30.7701, -59.1255) (-30.6972, -59.0781) (-30.7084, -58.8061) (-31.0276, -57.9695) (-30.1282, -57.2515) (-30.1477, -56.8484) (-28.7216, -55.8542) (-30.3416, -56.3459) (-30.8076, -56.6159) (-31.4332, -57.5286) (-31.8455, -58.3311) (-31.1035, -59.0517) (-30.8432, -59.1731) (-30.7701, -59.1255) knots 0 0 0 0 0 0 0.136568 0.224337 0.328745 0.437281 0.54436 0.65508 0.767311 0.862903 1 1 1 1 1 1
  spline S87 degree 5 poles (-32.5781, -60.807) (-32.5773, -60.7303) (-33.0278, -60.7608) (-34.7745, -61.1852) (-34.1977, -59.3622) (-38.6304, -61.4094) (-34.7501, -60.3343) (-35.3612, -62.2052) (-33.1231, -61.2208) (-32.579, -60.8915) (-32.5781, -60.807) knots 0 0 0 0 0 0 0.191347 0.318684 0.480917 0.65254 0.789187 1 1 1 1 1 1
  spline S88 degree 5 poles (-34.1278, -63.2232) (-34.2513, -63.0931) (-34.8215, -62.8819) (-36.3509, -62.751) (-37.0656, -63.9036) (-37.9761, -65.5302) (-39.0773, -65.641) (-39.7927, -67.2487) (-41.2874, -64.8465) (-39.3236, -64.8939) (-40.8672, -64.0221) (-41.5041, -65.618) (-40.9442, -66.0842) (-40.716, -67.124) (-39.1994, -67.1487) (-38.2376, -66.325) (-37.2703, -65.1909) (-36.1299, -63.9076) (-36.0571, -63.6983) (-34.5202, -63.6236) (-34.0609, -63.4379) (-34.056, -63.2988) (-34.1278, -63.2232) knots 0 0 0 0 0 0 0.082557 0.13669 0.201121 0.264553 0.321233 0.370931 0.419664 0.467875 0.513884 0.562809 0.617131 0.674986 0.735677 0.796507 0.858727 0.912778 0.952059 1 1 1 1 1 1
  spline S89 degree 5 poles (-33.1069, -64.1354) (-33.1569, -64.0176) (-33.624, -63.8178) (-35.3627, -63.7206) (-35.4325, -64.5574) (-37.3919, -65.9618) (-37.8536, -66.7514) (-39.4909, -67.564) (-40.8371, -67.3091) (-41.619, -67.1519) (-43.4168, -66.1357) (-44.0298, -69.8563) (-43.2358, -68.115) (-43.4047, -67.5957) (-41.908, -67.3014) (-41.6009, -67.439) (-40.4071, -68.312) (-39.8398, -68.505) (-38.6601, -69.122) (-36.4192, -66.2731) (-35.4801, -66.0563) (-34.6795, -64.1899) (-33.8771, -64.5054) (-33.185, -64.3475) (-33.0755, -64.2092) (-33.1069, -64.1354) knots 0 0 0 0 0 0 0.063707 0.107144 0.161317 0.21528 0.267686 0.318471 0.369518 0.416257 0.460739 0.504515 0.544593 0.58304 0.623006 0.663986 0.71182 0.764991 0.819177 0.874092 0.92481 0.960063 1 1 1 1 1 1
  spline S90 degree 5 poles (-32.5781, -64.9853) (-32.6549, -64.8983) (-32.9572, -64.8367) (-33.7955, -65.0531) (-33.7717, -65.83) (-35.0841, -66.1785) (-35.4288, -66.8397) (-37.2934, -67.3325) (-34.6097, -67.5162) (-34.1595, -66.8505) (-33.3618, -66.0593) (-32.9538, -65.7047) (-32.5254, -65.2611) (-32.5122, -65.0599) (-32.5781, -64.9853) knots 0 0 0 0 0 0 0.115782 0.198561 0.297578 0.401379 0.508958 0.616279 0.720837 0.82182 0.900621 1 1 1 1 1 1
  spline S91 degree 5 poles (-38.2478, -68.9176) (-38.2449, -68.8982) (-37.8672, -68.6989) (-36.2239, -67.4887) (-36.0119, -68.6965) (-33.6922, -67.5226) (-32.9845, -67.6703) (-31.3567, -64.5678) (-31.5973, -67.3447) (-32.7751, -67.9434) (-33.5759, -69.6324) (-34.9158, -68.9068) (-36.6648, -70.1638) (-37.5189, -68.7581) (-38.1234, -68.8913) (-38.2494, -68.9281) (-38.2478, -68.9176) knots 0 0 0 0 0 0 0.106962 0.1814 0.272854 0.360395 0.449551 0.536962 0.623945 0.715489 0.808432 0.884169 0.94191 1 1 1 1 1 1
  spline S92 degree 5 poles (-46.3881, -67.9862) (-46.433, -67.924) (-46.1005, -67.6532) (-44.5389, -66.8577) (-44.1124, -66.3985) (-41.7373, -64.201) (-41.5239, -63.0498) (-39.9523, -60.2592) (-39.414, -60.6595) (-35.2593, -57.3979) (-35.7147, -58.8772) (-36.9273, -59.598) (-38.5071, -60.705) (-39.4721, -61.1891) (-40.357, -64.3485) (-42.8785, -66.4467) (-42.6938, -67.0018) (-45.5858, -67.946) (-46.3311, -68.0654) (-46.3881, -67.9862) knots 0 0 0 0 0 0 0.069332 0.12174 0.18835 0.261254 0.336028 0.400686 0.461776 0.521198 0.577227 0.634424 0.702868 0.775301 0.849269 0.91178 1 1 1 1 1 1
  spline S93 degree 4 poles (-42.9668, -61.9713) (-43.5476, -62.014) (-44.8832, -63.1209) (-46.9868, -62.531) (-47.9555, -60.9144) (-47.2306, -59.4569) (-46.3922, -59.0501) (-45.0686, -58.5222) (-44.2052, -58.6659) knots 0 0 0 0 0 0.333147 0.462296 0.580047 0.69202 1 1 1 1 1
  spline S94 degree 4 poles (-42.9668, -61.9713) (-43.3729, -62.309) (-43.5671, -63.5547) (-46.0299, -64.6595) (-48.4477, -64.1223) (-50.5937, -63.1413) (-50.3441, -60.3816) (-49.5185, -59.2305) (-47.3592, -57.9055) (-45.6956, -58.321) (-43.9843, -58.1068) (-44.03, -58.7973) (-44.2052, -58.6659) knots 0 0 0 0 0 0.205585 0.305091 0.409552 0.511003 0.6133 0.715159 0.809989 0.889595 1 1 1 1 1
  spline S95 degree 5 poles (-42.304, -62.2589) (-42.2097, -62.3419) (-42.2389, -62.7895) (-42.9204, -64.1888) (-43.6254, -64.264) (-44.0888, -66.2178) (-50.2898, -69.3293) (-48.6353, -66.9397) (-47.5276, -67.3416) (-45.7763, -64.4659) (-44.4196, -64.3914) (-43.7604, -63.3341) (-42.7515, -62.3036) (-42.3969, -62.1771) (-42.304, -62.2589) knots 0 0 0 0 0 0 0.105213 0.195603 0.297105 0.40229 0.514222 0.621227 0.717438 0.815936 0.896385 1 1 1 1 1 1
  spline S96 degree 5 poles (-46.3881, -64.6916) (-46.6303, -64.609) (-47.4647, -64.8149) (-49.4188, -66.2428) (-50.7152, -66.4957) (-52.2222, -68.6825) (-56.0634, -67.353) (-55.3782, -68.8262) (-53.4139, -67.9111) (-52.59, -68.6415) (-50.5579, -67.6767) (-48.3878, -67.5151) (-47.981, -65.8139) (-46.476, -65.5007) (-46.1578, -64.9273) (-46.2601, -64.7353) (-46.3881, -64.6916) knots 0 0 0 0 0 0 0.128656 0.212007 0.302017 0.38736 0.464986 0.538167 0.615145 0.703798 0.791679 0.871489 0.931974 1 1 1 1 1 1
  spline S97 degree 5 poles (-47.7792, -64.8474) (-47.8135, -64.7652) (-48.3884, -64.6333) (-50.6778, -64.4267) (-51.2476, -65.4806) (-53.9982, -65.9285) (-57.0932, -67.0393) (-58.7992, -64.7564) (-65.9481, -66.213) (-61.1647, -65.7412) (-61.2741, -66.3201) (-57.5895, -67.323) (-56.4269, -67.1468) (-52.5338, -67.2788) (-51.4925, -66.8769) (-49.8915, -65.3295) (-48.1127, -65.061) (-47.7488, -64.9205) (-47.7792, -64.8474) knots 0 0 0 0 0 0 0.077589 0.135347 0.214261 0.295563 0.37314 0.447365 0.519488 0.585801 0.655733 0.728287 0.806154 0.876272 0.931045 1 1 1 1 1 1
  spline S98 degree 5 poles (-59.4622, -65.4066) (-59.4679, -65.329) (-58.8222, -65.2672) (-56.021, -65.3807) (-54.8023, -64.375) (-54.1102, -62.5377) (-47.2709, -64.4774) (-50.9616, -64.0732) (-51.0787, -64.4953) (-54.2869, -65.2407) (-54.434, -65.8955) (-56.488, -65.8685) (-57.4314, -65.9499) (-59.0337, -65.6192) (-59.4576, -65.4695) (-59.4622, -65.4066) knots 0 0 0 0 0 0 0.121242 0.208016 0.307031 0.404077 0.498704 0.585114 0.664461 0.751448 0.83695 0.901736 1 1 1 1 1 1
  spline S99 degree 5 poles (-62.0744, -65.1219) (-62.0334, -65.0084) (-61.6459, -64.8187) (-60.2226, -64.7206) (-59.2563, -63.8527) (-58.0609, -62.7487) (-55.7224, -62.2086) (-55.3357, -61.3792) (-49.396, -62.5) (-51.8191, -62.7473) (-53.8737, -62.3483) (-55.7408, -63.6017) (-57.3412, -63.7318) (-58.6338, -65.2611) (-59.9496, -64.622) (-61.2567, -65.5359) (-61.9818, -65.3586) (-62.1042, -65.2042) (-62.0744, -65.1219) knots 0 0 0 0 0 0 0.079636 0.137468 0.212555 0.296399 0.372212 0.449878 0.528404 0.605154 0.676705 0.755203 0.830412 0.894055 0.942217 1 1 1 1 1 1
  spline S100 degree 5 poles (-60.6291, -62.9598) (-60.6891, -62.8769) (-60.4504, -62.418) (-58.432, -60.9364) (-57.1576, -60.8714) (-55.8704, -59.1419) (-49.5511, -60.4959) (-50.9884, -61.5149) (-52.9353, -61.1739) (-54.0485, -61.1005) (-55.5539, -61.5557) (-56.8461, -60.9459) (-57.7531, -61.8761) (-58.3505, -62.1756) (-60.1412, -62.1936) (-60.1137, -62.7869) (-60.4711, -63) (-60.6014, -62.9981) (-60.6291, -62.9598) knots 0 0 0 0 0 0 0.101106 0.180306 0.26865 0.359773 0.444112 0.521813 0.589054 0.659381 0.727726 0.795985 0.858394 0.911954 0.953282 1 1 1 1 1 1
  spline S101 degree 5 poles (-60.1098, -60.41) (-60.1896, -60.3455) (-59.7051, -59.8494) (-57.1829, -57.9819) (-57.3638, -57.8466) (-46.3254, -57.3862) (-50.4282, -59.8665) (-51.1873, -59.0362) (-53.9757, -59.2496) (-54.8029, -58.6569) (-57.5142, -59.6403) (-58.0751, -59.6021) (-59.5906, -60.32) (-60.0495, -60.4589) (-60.1098, -60.41) knots 0 0 0 0 0 0 0.133387 0.226344 0.336387 0.451478 0.555941 0.645301 0.738205 0.828162 0.899017 1 1 1 1 1 1
  spline S102 degree 5 poles (-47.9233, -57.9066) (-47.8857, -57.7837) (-48.3084, -57.435) (-50.1297, -56.6156) (-50.093, -56.3706) (-53.0841, -55.5141) (-54.1936, -55.6592) (-55.6657, -56.1588) (-56.3493, -56.7417) (-57.5293, -57.8794) (-54.3487, -55.6792) (-53.9845, -56.929) (-51.8283, -56.8528) (-51.4162, -57.5879) (-50.3585, -57.8255) (-48.4664, -58.0932) (-47.9598, -58.026) (-47.9233, -57.9066) knots 0 0 0 0 0 0 0.099994 0.169331 0.253192 0.335339 0.407168 0.475152 0.543186 0.613092 0.68188 0.760877 0.840123 0.902752 1 1 1 1 1 1
  spline S103 degree 5 poles (-45.4747, -57.8009) (-45.4536, -57.7311) (-45.7791, -57.5777) (-47.1124, -57.3077) (-47.5165, -57.0031) (-48.3834, -55.9295) (-47.8608, -54.8152) (-49.7113, -53.9179) (-49.8111, -56.5906) (-48.0827, -57.0435) (-48.1816, -57.8806) (-46.0555, -57.9692) (-45.5, -57.8845) (-45.4747, -57.8009) knots 0 0 0 0 0 0 0.126081 0.209877 0.311715 0.417095 0.523875 0.634423 0.750628 0.848789 1 1 1 1 1 1
  spline S104 degree 4 poles (-29.9718, -31.3956) (-29.1247, -30.8166) (-30.0858, -32.3983) (-28.5656, -32.0793) (-28.9057, -32.8535) (-29.2923, -33.0416) (-29.0918, -33.4298) (-29.0564, -33.9315) (-29.6334, -33.713) (-29.632, -33.3693) (-30.1623, -33.2822) (-30.1943, -32.9223) (-29.9747, -32.5646) (-30.2458, -32.2645) (-30.4997, -32.0282) (-30.4031, -31.9459) knots 0 0 0 0 0 0.202828 0.279396 0.349203 0.415262 0.480988 0.546469 0.612539 0.677713 0.741261 0.803425 0.864654 1 1 1 1 1
  spline S105 degree 4 poles (-30.4031, -31.9459) (-30.3437, -31.5829) (-29.6758, -32.9406) (-29.8173, -31.3903) (-30.2039, -31.6136) (-29.9718, -31.3956) knots 0 0 0 0 0 0.507369 1 1 1 1 1
  spline S106 degree 5 poles (-37.084, -12.6167) (-37.0659, -12.5722) (-37.1594, -12.4592) (-37.6373, -12.247) (-38.0134, -12.3198) (-38.0318, -11.5374) (-38.7609, -11.5867) (-39.0848, -12.2883) (-38.422, -12.6705) (-38.0056, -12.2211) (-37.7964, -12.5996) (-37.2604, -12.6987) (-37.1025, -12.6621) (-37.084, -12.6167) knots 0 0 0 0 0 0 0.129633 0.218545 0.330734 0.445987 0.556865 0.669063 0.78015 0.867961 1 1 1 1 1 1
  spline S107 degree 5 poles (-36.7419, -12.2915) (-36.7048, -12.2726) (-36.7381, -12.1271) (-37.0523, -11.6569) (-37.4719, -11.5294) (-37.2628, -10.9516) (-37.6, -10.7558) (-37.9627, -10.701) (-38.2458, -11.0859) (-38.2128, -11.214) (-37.9708, -11.6419) (-37.4898, -11.5688) (-37.3668, -11.7886) (-36.9421, -12.2216) (-36.7803, -12.3111) (-36.7419, -12.2915) knots 0 0 0 0 0 0 0.121523 0.198728 0.292516 0.384284 0.464286 0.54256 0.622475 0.706615 0.796574 0.874261 1 1 1 1 1 1
  spline S108 degree 5 poles (-36.3513, -11.9711) (-36.3103, -11.9829) (-36.2616, -11.8738) (-36.2591, -11.4069) (-36.4126, -11.2664) (-36.3271, -10.903) (-36.0383, -10.5529) (-36.4468, -10.387) (-36.7355, -10.2778) (-37.0183, -10.5072) (-37.1092, -10.889) (-36.7533, -10.9935) (-36.6731, -11.0769) (-36.5017, -11.7634) (-36.3999, -11.9571) (-36.3513, -11.9711) knots 0 0 0 0 0 0 0.111769 0.185203 0.275341 0.365303 0.451719 0.536372 0.617658 0.699296 0.791849 0.86722 1 1 1 1 1 1
  spline S109 degree 5 poles (-35.8169, -12.1266) (-35.7658, -12.1406) (-35.6397, -12.0355) (-35.3985, -11.476) (-35.5176, -11.1834) (-34.8665, -11.1232) (-34.8125, -10.6296) (-35.2778, -10.2887) (-35.5614, -10.4253) (-35.905, -10.7387) (-35.5978, -11.0026) (-35.6318, -11.2028) (-35.7371, -11.7435) (-35.8732, -11.7561) (-35.8937, -12.0293) (-35.8538, -12.1165) (-35.8169, -12.1266) knots 0 0 0 0 0 0 0.11847 0.193632 0.287157 0.37685 0.46178 0.542723 0.621651 0.700965 0.778787 0.853647 0.914449 1 1 1 1 1 1
  spline S110 degree 5 poles (-35.3968, -12.3339) (-35.3716, -12.3631) (-35.2128, -12.3129) (-34.6482, -11.9165) (-34.8368, -11.6613) (-33.8881, -11.7606) (-34.0116, -11.4706) (-33.9952, -10.9253) (-34.4068, -10.9298) (-34.9135, -11.234) (-34.7065, -11.5273) (-34.8888, -11.6986) (-35.2422, -11.9868) (-35.2233, -12.0334) (-35.3872, -12.2366) (-35.4135, -12.3146) (-35.3968, -12.3339) knots 0 0 0 0 0 0 0.123304 0.198649 0.2917 0.380264 0.467816 0.548936 0.630514 0.711278 0.789258 0.860672 0.918303 1 1 1 1 1 1
  spline S111 degree 5 poles (-34.9284, -12.6167) (-34.9265, -12.582) (-34.7763, -12.519) (-34.1724, -12.414) (-34.1501, -11.9859) (-33.7516, -11.712) (-33.0499, -11.916) (-33.2487, -12.3348) (-33.3568, -12.6108) (-33.8258, -12.7466) (-34.003, -12.3466) (-34.2664, -12.6877) (-34.5021, -12.7392) (-34.8432, -12.6853) (-34.9299, -12.6438) (-34.9284, -12.6167) knots 0 0 0 0 0 0 0.127573 0.211589 0.312278 0.409585 0.500845 0.587217 0.668519 0.75307 0.835469 0.90066 1 1 1 1 1 1
  point P0 (0, 0)
  point P1 (-35.2849, -13.4961)
  point P2 (-35.2858, -13.8769)
  point P3 (-35.6774, -14.3506)
  point P4 (-35.7083, -14.6712)
  point P5 (-35.8193, -15.1642)
  point P6 (-36.3513, -15.5673)
  point P7 (-37.2047, -15.3482)
  point P8 (-37.084, -14.8755)
  point P9 (-36.8024, -14.1313)
  point P10 (-35.9678, -13.6284)
  point P11 (-35.8169, -13.4976)
  point P12 (-36.2788, -13.2161)
  point P13 (-36.6716, -13.1458)
  point P14 (-37.2045, -13.4275)
  point P15 (-37.8683, -14.2623)
  point P16 (-38.9139, -16.8675)
  point P17 (-38.1805, -15.76)
  point P18 (-38.5624, -16.9472)
  point P19 (-37.6472, -16.3841)
  point P20 (-36.742, -16.535)
  point P21 (-35.2838, -15.6399)
  point P22 (-35.0827, -16.0723)
  point P23 (-35.0198, -13.1457)
  point P24 (-33.1377, -15.7605)
  point P25 (-33.8477, -18.3174)
  point P26 (-34.1394, -18.7621)
  point P27 (-32.8367, -20.2244)
  point P28 (-32.2469, -20.9186)
  point P29 (-28.5742, -22.5572)
  point P30 (-26.7463, -23.6092)
  point P31 (-25.7864, -24.6744)
  point P32 (-25.362, -25.4898)
  point P33 (-25.7861, -25.0714)
  point P34 (-27.479, -23.6814)
  point P35 (-30.6736, -22.7008)
  point P36 (-31.8273, -22.7008)
  point P37 (-32.6443, -22.2683)
  point P38 (-35.706, -21.8356)
  point P39 (-37.2044, -23.6096)
  point P40 (-36.7419, -25.9933)
  point P41 (-35.5981, -26.9708)
  point P42 (-36.0568, -27.1155)
  point P43 (-37.3254, -26.2338)
  point P44 (-37.4336, -25.8053)
  point P45 (-38.1802, -25.071)
  point P46 (-38.3078, -23.2684)
  point P47 (-38.8048, -21.9486)
  point P48 (-38.4695, -19.7213)
  point P49 (-36.8024, -18.3174)
  point P50 (-32.1681, -23.1876)
  point P51 (-29.7346, -23.6092)
  point P52 (-28.5742, -25.1323)
  point P53 (-28.9042, -24.7959)
  point P54 (-29.682, -24.1179)
  point P55 (-30.6071, -23.8288)
  point P56 (-32.5255, -23.6092)
  point P57 (-33.5083, -22.5885)
  point P58 (-34.1278, -27.0517)
  point P59 (-33.1496, -26.7161)
  point P60 (-32.8272, -26.2336)
  point P61 (-31.5299, -26.5279)
  point P62 (-30.9763, -25.6937)
  point P63 (-30.3205, -25.6514)